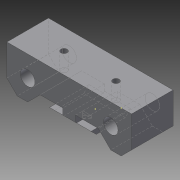
# Autodesk Inventor part: Moving block
Saved by Autodesk Inventor 2015 (Build 190159000, 159)
## iProperties
Created: 2019-01-17
Part Number: Moving block
Material: Generic
Document SubType Name: Modeling
Designer: Toby
Density: 1 g/cm^3
Appearance: Default
Author: Toby
Autodesk Inventor part; units mm, degrees
ref_plane "YZ Plane" through (0, 0, 0) normal (1, 0, 0) x (0, 1, 0)
ref_plane "XZ Plane" through (0, 0, 0) normal (0, 1, 0) x (-1, 0, 0)
ref_plane "XY Plane" through (0, 0, 0) normal (0, 0, 1) x (1, 0, 0)
sketch "Sketch1" plane through (0, 0, 0) normal (0, 0, 1) x (1, 0, 0)
  line L0 (-35.1442, 12.6555) -> (24.8558, 12.6555)
  line L1 (24.8558, 12.6555) -> (24.8558, -7.3445)
  line L2 (24.8558, -7.3445) -> (-35.1442, -7.3445)
  line L3 (-35.1442, -7.3445) -> (-35.1442, 12.6555)
  point P0 (0, 0)
  dimension "d0" = 60
  dimension "d1" = 20
  constraints: 8 end point, 2 parallel, 1 horizontal, 1 perpendicular
  measures "d0" distance of L0.start L0.end
  measures "d1" distance of L2.end L0.start
extrude "Extrusion1" add sketch "Sketch1" along normal blind 20
sketch "Sketch2" plane through (-35.1442, 12.6555, 0) normal (0, 1, 0) x (1, 0, 0)
  line L0 (0, 0) -> (0, -20) projected
  line L1 (60, 0) -> (60, -20) projected
  line L2 (0, 0) -> (60, 0) projected
  circle A0 centre (10, -10) radius 3.5
  circle A1 centre (50, -10) radius 3.5
  point P0 (35.1442, 0)
  dimension "d4" = 40
  dimension "d5" = 10
  dimension "d6" = 10
  dimension "d7" = 10
  dimension "d8" = 7
  dimension "d9" = 7
  constraints: 2 centre point, 2 coincident
  measures "d4" distance of point (50, -10) point (10, -10)
  measures "d5" distance from line of L0 point (10, -10)
  measures "d6" distance from line of L1 point (50, -10)
  measures "d7" distance from line of L2 point (50, -10)
  measures "d8" diameter of A0
  measures "d9" diameter of A1
extrude "Extrusion2" cut sketch "Sketch2" against normal blind 20
sketch "Sketch3" plane through (0, 0, 20) normal (0, 0, 1) x (1, 0, 0)
  line L0 (-35.1442, 12.6555) -> (24.8558, 12.6555) projected
  line L1 (-35.1442, 12.6555) -> (-35.1442, -7.3445) projected
  line L2 (24.8558, -7.3445) -> (24.8558, 12.6555) projected
  point P0 (0, 0)
  point P1 (-17.6442, 2.6555)
  point P2 (7.3558, 2.6555)
  dimension "d12" = 10
  dimension "d13" = 10
  dimension "d14" = 25
  dimension "d15" = 17.5
  dimension "d16" = 17.5
  measures "d12" distance from line of L0 point (-17.644, 2.656)
  measures "d13" distance from line of L0 point (7.356, 2.656)
  measures "d14" distance of point (7.356, 2.656) point (-17.644, 2.656)
  measures "d15" distance from line of L1 point (-17.644, 2.656)
  measures "d16" distance from line of L2 point (7.356, 2.656)
hole "Hole1" at (-17.6442, 2.6555, 20) at (7.3558, 2.6555, 20) direction (0, 0, -1) diameter 3 depth 8 tip angle 118
sketch "Sketch4" plane through (-35.1442, 12.6555, 0) normal (0, 1, 0) x (1, 0, 0)
  line L0 (60, 0) -> (0, 0) projected
  line L1 (16, 0) -> (44, 0)
  line L2 (44, 0) -> (44, -6)
  line L3 (44, -6) -> (16, -6)
  line L4 (16, -6) -> (16, 0)
  line L5 (0, 0) -> (0, -20) projected
  line L6 (60, 0) -> (60, -20) projected
  point P0 (35.1442, 0)
  dimension "d24" = 16
  dimension "d25" = 16
  dimension "d26" = 6
  constraints: 8 end point, 2 parallel, 1 horizontal, 1 perpendicular, 1 point on line
  measures "d24" distance between parallel lines of L5 L4
  measures "d25" distance between parallel lines of L6 L2
  measures "d26" distance between parallel lines of L0 L3
extrude "Extrusion3" cut sketch "Sketch4" against normal blind 20
chamfer "Chamfer1" distance 6 angle 45 2 edges at (8.8558, 2.6555, 0) (-19.1442, 2.6555, 0)
sketch "Sketch5" plane through (-35.1442, 12.6555, 20) normal (0, 1, 0) x (1, 0, 0)
  point P0 (35.1442, 20)
sketch "Sketch6" plane through (8.8558, 12.6555, 6) normal (0, 0, -1) x (-1, 0, 0)
  point P0 (8.8558, -12.6555)
sketch "Sketch7" plane through (-35.1442, 12.6555, 20) normal (0, 1, 0) x (1, 0, 0)
  line L0 (20, 20) -> (40, 20)
  line L1 (40, 20) -> (40, 17.5)
  line L2 (40, 17.5) -> (20, 17.5)
  line L3 (20, 17.5) -> (20, 20)
  line L4 (0, 20) -> (0, 0) projected
  line L5 (60, 20) -> (60, 0) projected
  line L6 (50, 20) -> (60, 20) projected
  line L7 (44, 14) -> (16, 14) projected
  line L8 (27, 14) -> (33, 14)
  line L9 (33, 14) -> (33, 17.5)
  line L10 (33, 17.5) -> (27, 17.5)
  line L11 (27, 17.5) -> (27, 14)
  point P0 (35.1442, 20)
  dimension "d32" = 20
  dimension "d33" = 20
  dimension "d34" = 2.5
  dimension "d35" = 7
  dimension "d36" = 7
  constraints: 16 end point, 4 parallel, 2 horizontal, 2 perpendicular, 2 point on line, 1 collinear
  measures "d32" distance between parallel lines of L4 L3
  measures "d33" distance between parallel lines of L5 L1
  measures "d34" distance between parallel lines of L0 L2
  measures "d35" distance between parallel lines of L3 L11
  measures "d36" distance between parallel lines of L1 L9
extrude "Extrusion4" add sketch "Sketch7" against normal blind 20
chamfer "Chamfer2" distance 3 angle 45 2 edges at (-5.1442, 12.6555, 0) (-5.1442, -7.3445, 0)
chamfer "Chamfer3" distance 5 angle 45 2 edges at (24.8558, 2.6555, 0) (-35.1442, 2.6555, 0)
sketch "Sketch8" plane through (4.8558, -4.3445, 0) normal (0, 0, -1) x (-1, 0, 0)
  line L0 (10, 3.5052) -> (12.1213, 5.6266)
  line L1 (10, 3.5052) -> (13, 3.5052) construction
  line L2 (12.1213, 5.6266) -> (7.8787, 5.6266)
  line L3 (7.8787, 5.6266) -> (10, 3.5052)
  point P0 (4.8558, 4.3445)
  dimension "d45" = 3
  dimension "d46" = 45
  constraints: 8 end point, 2 horizontal, 1 equal length, 1 perpendicular
  measures "d45" distance of L0.start L0.end
  measures "d46" angle of L1 L0
extrude "Extrusion5" cut sketch "Sketch8" against normal blind 1
body "Solid1"
